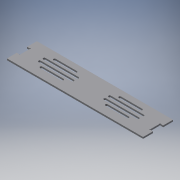
# Autodesk Inventor part: placa auto falante
Saved by Autodesk Inventor 2016 (Build 200138000, 138)
## iProperties
Created: 2017-06-08
Part Number: placa auto falante
Material: Genérico
Document SubType Name: Modeling
Designer: Fabio
Density: 1 g/cm^3
Appearance: Padrão
Author: Fabio
Autodesk Inventor part; units mm, degrees
ref_plane "YZ Plane" through (0, 0, 0) normal (1, 0, 0) x (0, 1, 0)
ref_plane "XZ Plane" through (0, 0, 0) normal (0, 1, 0) x (-1, 0, 0)
ref_plane "XY Plane" through (0, 0, 0) normal (0, 0, 1) x (1, 0, 0)
sketch "Esboço1" plane through (0, 0, 0) normal (0, 0, 1) x (1, 0, 0)
  line L0 (-173, 38) -> (173, 38)
  line L1 (173, 38) -> (173, -38)
  line L2 (173, -38) -> (-173, -38)
  line L3 (-173, -38) -> (-173, 38)
  point P0 (0, 0)
  point P1 (173, 0)
  point P2 (0, 38)
  dimension "d0" = 346
  dimension "d1" = 76
  constraints: 8 end point, 2 midpoint, 2 parallel, 1 horizontal, 1 horizontal alignment, 1 perpendicular, 1 vertical alignment
  measures "d0" distance between parallel lines of L3 L1
  measures "d1" distance between parallel lines of L2 L0
extrude "Extrusão1" add sketch "Esboço1" along normal blind 4
sketch "Esboço2" plane through (0, 0, 4) normal (0, 0, 1) x (1, 0, 0)
  line L0 (-173, 38) -> (-173, -38) projected
  line L1 (-173, 13) -> (-165, 13)
  line L2 (-165, 13) -> (-165, -13)
  line L3 (-165, -13) -> (-173, -13)
  line L4 (-173, -13) -> (-173, 13)
  line L5 (173, 38) -> (-173, 38) projected
  circle A0 centre (-165, 13) radius 1
  circle A1 centre (-165, -13) radius 1
  point P0 (0, 0)
  dimension "d4" = 8
  dimension "d5" = 26
  dimension "d6" = 25
  dimension "d7" = 2
  dimension "d8" = 2
  constraints: 8 end point, 2 centre point, 2 coincident, 2 parallel, 1 horizontal, 1 perpendicular, 1 point on line
  measures "d4" distance of L2.end L3.end
  measures "d5" distance between parallel lines of L1 L3
  measures "d6" distance between parallel lines of L5 L1
  measures "d7" diameter of A0
  measures "d8" diameter of A1
extrude "Extrusão2" cut sketch "Esboço2" against normal blind 10
mirror "Espelhamento1" about plane through (0, 0, 0) normal (1, 0, 0) of "Extrusão2"
sketch "Esboço3" plane through (0, 0, 0) normal (0, 0, -1) x (-1, 0, 0)
  line L0 (-113, -17) -> (-38, -17)
  line L1 (173, 38) -> (-173, 38) projected
  line L2 (-165, 12) -> (-165, -12) projected
  line L3 (-56, 23) -> (-110, 23)
  line L4 (-113, 20) -> (-113, 20)
  line L5 (-110, 17) -> (-56, 17)
  line L6 (-53, 20) -> (-53, 20)
  line L7 (-125, 12) -> (-41, 12)
  line L8 (-38, 9) -> (-38, 9)
  line L9 (-41, 6) -> (-125, 6)
  line L10 (-128, 9) -> (-128, 9)
  line L11 (-125, 0) -> (-41, 0)
  line L12 (-38, -3) -> (-38, -3)
  line L13 (-41, -6) -> (-125, -6)
  line L14 (-128, -3) -> (-128, -3)
  line L15 (-110, -17) -> (-56, -17)
  line L16 (-53, -14) -> (-53, -14)
  line L17 (-56, -11) -> (-110, -11)
  line L18 (-113, -14) -> (-113, -14)
  arc A0 (-113, -14) -> (-110, -17) centre (-110, -14) ccw
  arc A1 (-110, -11) -> (-113, -14) centre (-110, -14) ccw
  arc A2 (-56, -17) -> (-53, -14) centre (-56, -14) ccw
  arc A3 (-53, -14) -> (-56, -11) centre (-56, -14) ccw
  arc A4 (-38, -3) -> (-41, 0) centre (-41, -3) ccw
  arc A5 (-41, -6) -> (-38, -3) centre (-41, -3) ccw
  arc A6 (-41, 6) -> (-38, 9) centre (-41, 9) ccw
  arc A7 (-38, 9) -> (-41, 12) centre (-41, 9) ccw
  arc A8 (-56, 17) -> (-53, 20) centre (-56, 20) ccw
  arc A9 (-113, 20) -> (-110, 17) centre (-110, 20) ccw
  arc A10 (-110, 23) -> (-113, 20) centre (-110, 20) ccw
  arc A11 (-53, 20) -> (-56, 23) centre (-56, 20) ccw
  arc A12 (-128, -3) -> (-125, -6) centre (-125, -3) ccw
  arc A13 (-125, 0) -> (-128, -3) centre (-125, -3) ccw
  arc A14 (-128, 9) -> (-125, 6) centre (-125, 9) ccw
  arc A15 (-125, 12) -> (-128, 9) centre (-125, 9) ccw
  point P0 (0, 0)
  point P1 (-53, 23)
  point P2 (-38, 6)
  point P3 (-38, 12)
  point P4 (-38, -6)
  point P5 (-38, 0)
  point P6 (-53, -11)
  point P7 (-53, -17)
  dimension "d16" = 6
  dimension "d17" = 5
  dimension "d18" = 6
  dimension "d19" = 6
  dimension "d20" = 6
  dimension "d22" = 90
  dimension "d23" = 90
  dimension "d24" = 60
  dimension "d25" = 15
  dimension "d26" = 37
  dimension "d27" = 37
  dimension "d28" = 60
  dimension "d29" = 15
  dimension "d30" = 3
  dimension "d31" = 3
  dimension "d32" = 3
  dimension "d35" = 15
  dimension "d36" = 6
  dimension "d37" = 6
  dimension "d38" = 6
  dimension "d39" = 5
  constraints: 34 end point, 32 point on circle, 32 tangent, 16 centre point, 16 point on line, 13 equal radius, 8 parallel, 5 horizontal, 4 perpendicular
  measures "d16" distance of point (-38, 12) point (-38, 6)
  measures "d17" distance between parallel lines of L5 L7
  measures "d18" distance of point (-38, 0) point (-38, -6)
  measures "d19" distance between parallel lines of L9 L11
  measures "d20" distance of point (-53, -11) point (-53, -17)
  measures "d22" distance between parallel lines of L8 L10
  measures "d23" distance between parallel lines of L14 L12
  measures "d24" distance between parallel lines of L16 L18
  measures "d25" distance between parallel lines of L12 L16
  measures "d26" distance between parallel lines of L2 L10
  measures "d27" distance between parallel lines of L2 L14
  measures "d28" distance between parallel lines of L4 L6
  measures "d29" distance between parallel lines of L8 L6
  measures "d30" radius of A0
  measures "d31" radius of A11
  measures "d32" radius of A12
  measures "d35" distance between parallel lines of L1 L3
  measures "d36" distance between parallel lines of L5 L3
  measures "d37" distance between parallel lines of L9 L7
  measures "d38" distance between parallel lines of L15 L17
  measures "d39" distance between parallel lines of L13 L17
extrude "Extrusão3" cut sketch "Esboço3" against normal blind 10
mirror "Espelhamento2" about plane through (0, 0, 0) normal (1, 0, 0) of "Extrusão3"
